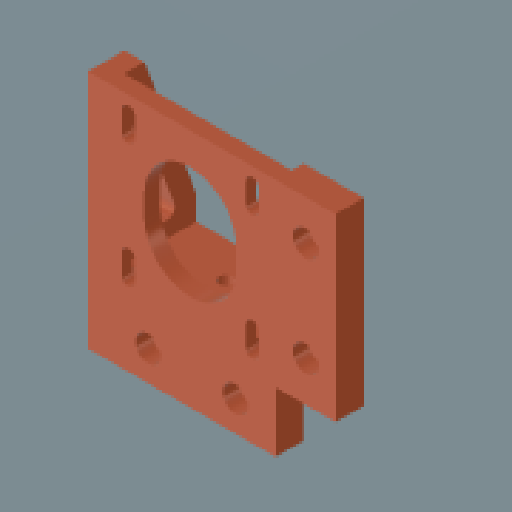
# Autodesk Inventor part: Alpha Motor Mount
Saved by Autodesk Inventor 2023.2 (Build 272271000, 271)
## iProperties
Created: 2023-02-03
Part Number: Alpha Motor Mount
Material: ABS Plastic
Document SubType Name: Modeling
Designer: remop
Density: 1.06 g/cm^3
Appearance: Smooth - Light Orange
Author: remop
Autodesk Inventor part; units mm, degrees
ref_plane "YZ Plane" through (0, 0, 0) normal (1, 0, 0) x (0, 1, 0)
ref_plane "XZ Plane" through (0, 0, 0) normal (0, 1, 0) x (-1, 0, 0)
ref_plane "XY Plane" through (0, 0, 0) normal (0, 0, 1) x (1, 0, 0)
sketch "Sketch1" plane through (0, 0, 0) normal (0, 0, 1) x (1, 0, 0)
  line L0 (0, 0) -> (0, 15)
  line L1 (0, 15) -> (15, 15)
  line L2 (15, 15) -> (15, 60)
  line L3 (15, 60) -> (-65, 60)
  line L4 (-65, 60) -> (-65, 0)
  line L5 (-65, 0) -> (0, 0)
  line L6 (-36.8, 25) -> (-36.8, 20) construction
  line L7 (-38.4, 25) -> (-38.4, 20)
  line L8 (-35.2, 20) -> (-35.2, 25)
  arc A0 (-35.2, 25) -> (-38.4, 25) centre (-36.8, 25) ccw
  arc A1 (-38.4, 20) -> (-35.2, 20) centre (-36.8, 20) ccw
  line L9 (-5.8, 25) -> (-5.8, 20) construction
  line L10 (-7.4, 25) -> (-7.4, 20)
  line L11 (-4.2, 20) -> (-4.2, 25)
  arc A2 (-4.2, 25) -> (-7.4, 25) centre (-5.8, 25) ccw
  arc A3 (-7.4, 20) -> (-4.2, 20) centre (-5.8, 20) ccw
  line L12 (-5.8, 56) -> (-5.8, 51) construction
  line L13 (-7.4, 56) -> (-7.4, 51)
  line L14 (-4.2, 51) -> (-4.2, 56)
  arc A4 (-4.2, 56) -> (-7.4, 56) centre (-5.8, 56) ccw
  arc A5 (-7.4, 51) -> (-4.2, 51) centre (-5.8, 51) ccw
  line L15 (-36.8, 56) -> (-36.8, 51) construction
  line L16 (-38.4, 56) -> (-38.4, 51)
  line L17 (-35.2, 51) -> (-35.2, 56)
  arc A6 (-35.2, 56) -> (-38.4, 56) centre (-36.8, 56) ccw
  arc A7 (-38.4, 51) -> (-35.2, 51) centre (-36.8, 51) ccw
  line L18 (-21.3, 40.5) -> (-21.3, 35.5) construction
  line L19 (-32.8, 40.5) -> (-32.8, 35.5)
  line L20 (-9.8, 35.5) -> (-9.8, 40.5)
  arc A8 (-9.8, 40.5) -> (-32.8, 40.5) centre (-21.3, 40.5) ccw
  arc A9 (-32.8, 35.5) -> (-9.8, 35.5) centre (-21.3, 35.5) ccw
  line L21 (-41.8, 60) -> (-41.8, 41)
  line L22 (-41.8, 41) -> (-55, 41)
  line L23 (-55, 41) -> (-65, 31)
  line L24 (-41.8, 41) -> (-41.8, 0)
  point P0 (-36.8, 22.5)
  point P1 (-5.8, 22.5)
  point P2 (-5.8, 53.5)
  point P3 (-36.8, 53.5)
  point P4 (-21.3, 38)
  dimension "d0" = 15
  dimension "d57" = 3.2
  dimension "d58" = 31
  dimension "d59" = 31
  dimension "d60" = 36.3
  dimension "d61" = 11.5
  dimension "d62" = 5
  dimension "d63" = 15.5
  dimension "d64" = 15.5
  dimension "d65" = 60
  dimension "d66" = 80
  dimension "d67" = 38
  dimension "d68" = 45
  dimension "d69" = 31
  dimension "d70" = 19
  dimension "d71" = 5
  constraints: 60 end point, 20 point on circle, 20 tangent, 10 centre point, 7 parallel, 7 perpendicular, 5 equal length, 5 midpoint, 5 point on line, 4 vertical, 3 equal radius, 2 horizontal alignment, 2 vertical alignment
  measures "d0" distance of L0.start L0.end
  measures "d57" distance between parallel lines of L8 L7
  measures "d58" distance of point (-5.8, 22.5) point (-36.8, 22.5)
  measures "d59" distance of point (-36.8, 53.5) point (-36.8, 22.5)
  measures "d60" distance from line of L2 point (-21.3, 38)
  measures "d61" radius of A9
  measures "d62" distance of L19.start L19.end
  measures "d63" distance from line of L18 point (-36.8, 22.5)
  measures "d64" horizontal distance of point (-36.8, 22.5) point (-21.3, 38)
  measures "d65" distance of L3.end L4.end
  measures "d66" distance of L2.end L3.end
  measures "d67" distance from line of L5 point (-21.3, 38)
  measures "d68" angle of L4 L23
  measures "d69" distance from line of L5 L23.end
  measures "d70" distance of L21.start L21.end
  measures "d71" distance from line of point (-36.8, 53.5) L21
extrude "Extrusion1" add sketch "Sketch1" along normal blind 4 contours L5 L24 L21 L3 L2 L1 L0
sketch "Sketch2" plane through (0, 0, 0) normal (0, 0, -1) x (-1, 0, 0)
  line L0 (0, 15) -> (-15, 15) projected
  line L1 (0, 0) -> (0, 15) projected
  line L2 (41.8, 0) -> (0, 0) projected
  line L3 (-15, 60) -> (41.8, 60) projected
  line L4 (-15, 15) -> (-15, 60) projected
  line L5 (0, 15) -> (-15, 15) projected
  line L6 (0, 15) -> (0, 60)
  line L7 (-15, 60) -> (41.8, 60) projected
  line L8 (41.8, 60) -> (41.8, 0) projected
  line L9 (0, 15) -> (41.8, 15)
  point P0 (65, 60)
  constraints: 4 end point, 2 point on line, 1 perpendicular, 1 vertical
extrude "Extrusion2" add sketch "Sketch2" along normal blind 3 contours L9 L8 L2 L1 | L0 L4 L3 L6
sketch "Sketch3" plane through (0, 0, 4) normal (0, 0, 1) x (1, 0, 0)
  line L0 (-41.8, 0) -> (0, 0) projected
  line L1 (0, 0) -> (0, 15) projected
  line L2 (0, 15) -> (15, 15) projected
  line L3 (15, 15) -> (15, 60) projected
  line L4 (15, 60) -> (-41.8, 60) projected
  line L5 (0, 60) -> (15, 60) projected
  line L6 (-41.8, 60) -> (-41.8, 0) projected
  line L7 (-41.8, 60) -> (-41.8, 0) projected
  point P0 (-10, 7.5)
  point P1 (-31.8, 7.5)
  point P2 (7.5, 25)
  point P3 (7.5, 50)
  point P4 (0, 7.5)
  point P5 (7.5, 15)
  point P6 (7.5, 60)
  dimension "d18" = 10
  dimension "d20" = 10
  dimension "d21" = 10
  dimension "d85" = 10
  constraints: 3 midpoint, 2 horizontal alignment, 2 vertical alignment
  measures "d18" distance from line of L1 point (-10, 7.5)
  measures "d20" distance from line of L2 point (7.5, 25)
  measures "d21" distance from line of L5 point (7.5, 50)
  measures "d85" distance from line of L6 point (-31.8, 7.5)
hole "Hole1" at (-10, 7.5, 4) at (-31.8, 7.5, 4) at (7.5, 25, 4) at (7.5, 50, 4) direction (0, 0, -1) diameter 3.6 end through all counterbore diameter 6.5 counterbore depth 4 clearance for "Socket Head Cap Screw ISO 4762" size "M3" standard "ISO"
sketch "Sketch9" plane through (-41.8, 40.5, 0) normal (-1, 0, 0) x (0, 0, 1)
  line L0 (4, 19.5) -> (4, -40.5) projected
  line L1 (0, 19.5) -> (4, 19.5) projected
  line L2 (0, -25.5) -> (-18, -25.5)
  line L3 (-18, -25.5) -> (-18, -15.5)
  line L4 (-18, -15.5) -> (-5, 19.5)
  line L5 (-5, 19.5) -> (0, 19.5)
  line L6 (4, 19.5) -> (-3, 19.5) projected
  line L7 (-13.4091, -17.5) -> (-3, 10.5245)
  line L8 (-3, 10.5245) -> (-3, -17.5)
  line L9 (-3, -17.5) -> (-13.4091, -17.5)
  line L10 (-3, -40.5) -> (4, -40.5) projected
  line L11 (0, 19.5) -> (0, -25.5) projected
  line L12 (-9, -25.5) -> (-3, -25.5) projected
  line L13 (0, -25.5) -> (-3, -25.5) projected
  line L14 (-3, -40.5) -> (-3, -25.5) projected
  point P0 (0, -40.5)
  point P1 (-9, 19)
  point P2 (0, -25.5)
  dimension "d75" = 10
  dimension "d76" = 5
  dimension "d77" = 5
  dimension "d86" = 8
  dimension "d87" = 3
  dimension "d94" = 15
  constraints: 14 end point, 2 coincident, 2 horizontal, 2 vertical, 1 collinear, 1 horizontal alignment, 1 parallel, 1 vertical alignment
  measures "d75" distance of L2.end L3.end
  measures "d76" distance of L4.end L5.end
  measures "d77" distance between parallel lines of L4 L7
  measures "d86" distance between parallel lines of L2 L9
  measures "d87" distance between parallel lines of L11 L8
  measures "d94" distance between parallel lines of L3 L14
extrude "Extrusion6" add sketch "Sketch9" along normal blind 5
sketch "Sketch10" plane through (0, 0, 0) normal (0, 0, -1) x (-1, 0, 0)
  line L0 (41.8, 60) -> (41.8, 15) projected
  line L1 (0, 60) -> (41.8, 60) projected
  line L2 (0, 60) -> (0, 15) projected
  arc A0 (32.8, 40.5) -> (9.8, 40.5) centre (21.3, 40.5) ccw projected
  line L3 (32.8, 35.5) -> (32.8, 40.5) projected
  arc A1 (9.8, 35.5) -> (32.8, 35.5) centre (21.3, 35.5) ccw projected
  line L4 (9.8, 40.5) -> (9.8, 35.5) projected
  arc A2 (38.4, 56) -> (35.2, 56) centre (36.8, 56) ccw projected
  line L5 (38.4, 51) -> (38.4, 56) projected
  arc A3 (35.2, 51) -> (38.4, 51) centre (36.8, 51) ccw projected
  line L6 (35.2, 56) -> (35.2, 51) projected
  arc A4 (7.4, 56) -> (4.2, 56) centre (5.8, 56) ccw projected
  line L7 (7.4, 51) -> (7.4, 56) projected
  arc A5 (4.2, 51) -> (7.4, 51) centre (5.8, 51) ccw projected
  line L8 (4.2, 56) -> (4.2, 51) projected
  arc A6 (7.4, 25) -> (4.2, 25) centre (5.8, 25) ccw projected
  line L9 (7.4, 20) -> (7.4, 25) projected
  arc A7 (4.2, 20) -> (7.4, 20) centre (5.8, 20) ccw projected
  line L10 (4.2, 25) -> (4.2, 20) projected
  arc A8 (38.4, 25) -> (35.2, 25) centre (36.8, 25) ccw projected
  line L11 (38.4, 20) -> (38.4, 25) projected
  arc A9 (35.2, 20) -> (38.4, 20) centre (36.8, 20) ccw projected
  line L12 (35.2, 25) -> (35.2, 20) projected
  line L13 (36.8, 56) -> (36.8, 51) construction
  line L14 (40.05, 56) -> (40.05, 51)
  line L15 (33.55, 51) -> (33.55, 56)
  arc A10 (40.05, 56) -> (33.55, 56) centre (36.8, 56) ccw
  arc A11 (33.55, 51) -> (40.05, 51) centre (36.8, 51) ccw
  line L16 (5.8, 51) -> (5.8, 56) construction
  line L17 (2.55, 51) -> (2.55, 56)
  line L18 (9.05, 56) -> (9.05, 51)
  arc A12 (2.55, 51) -> (9.05, 51) centre (5.8, 51) ccw
  arc A13 (9.05, 56) -> (2.55, 56) centre (5.8, 56) ccw
  line L19 (5.8, 20) -> (5.8, 25) construction
  line L20 (2.55, 20) -> (2.55, 25)
  line L21 (9.05, 25) -> (9.05, 20)
  arc A14 (2.55, 20) -> (9.05, 20) centre (5.8, 20) ccw
  arc A15 (9.05, 25) -> (2.55, 25) centre (5.8, 25) ccw
  line L22 (36.8, 20) -> (36.8, 25) construction
  line L23 (40.05, 20) -> (40.05, 25)
  line L24 (33.55, 25) -> (33.55, 20)
  arc A16 (33.55, 20) -> (40.05, 20) centre (36.8, 20) ccw
  arc A17 (40.05, 25) -> (33.55, 25) centre (36.8, 25) ccw
  line L25 (0, 15) -> (41.8, 15) projected
  point P0 (0, 0)
  point P1 (36.8, 53.5)
  point P2 (5.8, 53.5)
  point P3 (5.8, 22.5)
  point P4 (36.8, 22.5)
  dimension "d82" = 6.5
  constraints: 32 end point, 16 point on circle, 16 tangent, 8 centre point, 7 parallel, 4 midpoint, 3 equal radius, 1 vertical
  measures "d82" distance between parallel lines of L24 L23
extrude "Extrusion7" cut sketch "Sketch10" against normal blind 1.5 contours L14 A11 L15 A10 | L17 A13 L18 A12 | L20 A15 L21 A14 | A16 L24 A17 L23
sketch "Sketch11" plane through (0, 0, 0) normal (0, 0, -1) x (-1, 0, 0)
  arc A0 (2.55, 51) -> (9.05, 51) centre (5.8, 51) ccw projected
  line L0 (2.55, 51) -> (2.55, 56) projected
  arc A1 (9.05, 56) -> (2.55, 56) centre (5.8, 56) ccw projected
  line L1 (9.05, 56) -> (9.05, 51) projected
  arc A2 (2.55, 20) -> (9.05, 20) centre (5.8, 20) ccw projected
  line L2 (2.55, 20) -> (2.55, 25) projected
  arc A3 (9.05, 25) -> (2.55, 25) centre (5.8, 25) ccw projected
  line L3 (9.05, 25) -> (9.05, 20) projected
  arc A4 (40.05, 56) -> (33.55, 56) centre (36.8, 56) ccw projected
  line L4 (40.05, 56) -> (40.05, 51) projected
  arc A5 (33.55, 51) -> (40.05, 51) centre (36.8, 51) ccw projected
  line L5 (33.55, 51) -> (33.55, 56) projected
  line L6 (33.55, 20) -> (33.55, 25) projected
  arc A6 (40.05, 25) -> (33.55, 25) centre (36.8, 25) ccw projected
  line L7 (40.05, 25) -> (40.05, 20) projected
  arc A7 (33.55, 20) -> (40.05, 20) centre (36.8, 20) ccw projected
  arc A8 (32.8, 40.5) -> (9.8, 40.5) centre (21.3, 40.5) ccw projected
  line L8 (32.8, 35.5) -> (32.8, 40.5) projected
  arc A9 (9.8, 35.5) -> (32.8, 35.5) centre (21.3, 35.5) ccw projected
  line L9 (9.8, 40.5) -> (9.8, 35.5) projected
  line L10 (0, 60) -> (0, 15) projected
  line L11 (41.8, 60) -> (41.8, 15) projected
  line L12 (0, 60) -> (41.8, 60) projected
  line L13 (41.8, 60) -> (41.8, 15) projected
  line L14 (41.8, 19) -> (39.8923, 19)
  arc A10 (33.55, 20) -> (40.05, 20) centre (36.8, 20) ccw projected
  line L15 (33.7077, 19) -> (8.8923, 19)
  arc A11 (2.55, 20) -> (9.05, 20) centre (5.8, 20) ccw projected
  line L16 (2.7077, 19) -> (0, 19)
  line L17 (0, 0) -> (0, 15) projected
  line L18 (41.8, 15) -> (46.8, 15) projected
  line L19 (0, 15) -> (41.8, 15)
  line L20 (41.8, 15) -> (41.8, 19)
  line L21 (8.8923, 19) -> (8.8923, 15)
  line L22 (41.8, 51.0245) -> (41.8, 23) projected
  line L23 (0, 15) -> (41.8, 15) projected
  constraints: 12 end point, 7 point on line, 4 point on circle, 3 perpendicular, 1 horizontal
extrude "Extrusion8" add sketch "Sketch11" along normal up to surface (18 mm away) contours L15 A7 L14 L11 L19 L21
sketch "Sketch12" plane through (-46.8, 15, -18) normal (0, 0, -1) x (-1, 0, 0)
  line L0 (-37.9077, 0) -> (0, 0) projected
  line L1 (0, 10) -> (0, 0) projected
  line L2 (-5, 10) -> (0, 10) projected
  arc A0 (-13.0923, 4) -> (-6.9077, 4) centre (-10, 5) ccw projected
  line L3 (-37.9077, 4) -> (-13.0923, 4) projected
  line L4 (-37.9077, 0) -> (-37.9077, 4) projected
  arc A1 (-13.25, 5) -> (-13.0923, 4) centre (-10, 5) ccw projected
  line L5 (-13.0923, 4) -> (-6.9077, 4)
  arc A2 (-13.25, 5) -> (-6.75, 5) centre (-10, 5) ccw projected
  line L6 (-5, 10) -> (-5, 4) projected
  line L7 (-6.9077, 4) -> (-5, 4) projected
  point P0 (-46.8, -15)
  constraints: 2 end point, 1 horizontal, 1 point on circle
extrude "Extrusion9" add sketch "Sketch12" against normal blind 15 contours L5 A0
fillet "Fillet2" radius 2 3 edges at (-44.3, 51.0245, -3) (-44.3, 23, -13.4091) (-44.3, 23, -3)
sketch "Sketch13" plane through (-33.7077, 19, 0) normal (0, 1, 0) x (1, 0, 0)
  line L0 (24.8153, 18) -> (-8.0923, 18) projected
  line L1 (-8.0923, 0) -> (-8.0923, 18) projected
  line L2 (-6.1847, 0) -> (-8.0923, 0) projected
  line L3 (-6.1847, 0) -> (-6.1847, 3) projected
  line L4 (0, 3) -> (-6.1847, 3) projected
  line L5 (0, 0) -> (0, 3) projected
  line L6 (24.8153, 0) -> (0, 0) projected
  line L7 (24.8153, 0) -> (24.8153, 18) projected
  point P0 (33.7077, 0)
  point P1 (8.3615, 9)
  point P2 (8.3615, 18)
  point P3 (24.8153, 9)
  constraints: 2 midpoint, 1 horizontal alignment, 1 vertical alignment
hole "Hole2" at (-25.3462, 19, -9) direction (0, -1, 0) diameter 3.5 end through all
equation "\"d59\" = d58"
equation "\"d63\" = 0.5 * d58"
equation "\"d64\" = 0.5 * d59"
equation "\"d20\" = d18"
equation "\"d21\" = d20"
equation "\"d85\" = d18"
body "Solid1"
